Autodesk Fusion 360 part; units mm, degrees
(part 22 of 25)
  line L221 (7.4676, 44.45) -> (8.7884, 44.45)
  arc A279 (8.7884, 33.9598) -> (8.7884, 34.6202) centre (8.7884, 34.29) ccw
  arc A280 (2.3876, 44.7802) -> (2.3876, 44.1198) centre (2.3876, 44.45) ccw
  arc A281 (32.5501, 16.51) -> (33.4899, 16.51) centre (33.02, 16.51) ccw
  arc A282 (8.7884, 44.1198) -> (8.7884, 44.7802) centre (8.7884, 44.45) ccw
  arc A283 (3.7084, 44.1198) -> (3.7084, 44.7802) centre (3.7084, 44.45) ccw
  arc A284 (8.7884, 41.5798) -> (8.7884, 42.2402) centre (8.7884, 41.91) ccw
  arc A285 (3.7084, 41.5798) -> (3.7084, 42.2402) centre (3.7084, 41.91) ccw
  arc A286 (8.7884, 33.9598) -> (8.7884, 34.6202) centre (8.7884, 34.29) ccw
  arc A287 (2.3876, 42.2402) -> (2.3876, 41.5798) centre (2.3876, 41.91) ccw
  line L222 (4.6482, 3.971) -> (4.8936, 4.2164)
  arc A288 (3.7084, 41.5798) -> (3.7084, 42.2402) centre (3.7084, 41.91) ccw
  line L223 (4.6482, 6.511) -> (4.8936, 6.7564)
  line L224 (2.3876, 41.91) -> (3.7084, 41.91)
  line L225 (7.4676, 44.45) -> (8.7884, 44.45)
  arc A289 (7.4676, 42.2402) -> (7.4676, 41.5798) centre (7.4676, 41.91) ccw
  arc A290 (38.5699, 16.51) -> (37.6301, 16.51) centre (38.1, 16.51) ccw
  line L226 (4.8936, 5.9182) -> (4.6482, 6.1636)
  arc A291 (7.4676, 44.7802) -> (7.4676, 44.1198) centre (7.4676, 44.45) ccw
  line L227 (5.4864, 3.6236) -> (5.241, 3.3782)
  arc A292 (8.7884, 44.1198) -> (8.7884, 44.7802) centre (8.7884, 44.45) ccw
  arc A293 (7.4676, 34.6202) -> (7.4676, 33.9598) centre (7.4676, 34.29) ccw
  arc A294 (7.4676, 42.2402) -> (7.4676, 41.5798) centre (7.4676, 41.91) ccw
  arc A295 (8.7884, 41.5798) -> (8.7884, 42.2402) centre (8.7884, 41.91) ccw
  arc A296 (2.3876, 42.2402) -> (2.3876, 41.5798) centre (2.3876, 41.91) ccw
  line L228 (4.6482, 3.6236) -> (4.6482, 3.971)
  line L229 (5.4864, 3.6236) -> (5.241, 3.3782)
  line L230 (5.4864, 3.971) -> (5.4864, 3.6236)
  line L231 (5.241, 5.9182) -> (4.8936, 5.9182)
  line L232 (2.3876, 41.91) -> (3.7084, 41.91)
  line L233 (5.241, 5.9182) -> (4.8936, 5.9182)
  arc A297 (7.4676, 44.7802) -> (7.4676, 44.1198) centre (7.4676, 44.45) ccw
  line L234 (7.4676, 34.29) -> (8.7884, 34.29)
  line L235 (5.241, 6.7564) -> (5.4864, 6.511)
  line L236 (4.8936, 4.2164) -> (5.241, 4.2164)
  line L237 (4.6482, 6.1636) -> (4.6482, 6.511)
  line L238 (4.8936, 5.9182) -> (4.6482, 6.1636)
  arc A298 (41.1099, 16.51) -> (40.1701, 16.51) centre (40.64, 16.51) ccw
  arc A299 (41.1099, 16.51) -> (40.1701, 16.51) centre (40.64, 16.51) ccw
  arc A300 (2.3876, 44.7802) -> (2.3876, 44.1198) centre (2.3876, 44.45) ccw
  arc A301 (2.3876, 34.6202) -> (2.3876, 33.9598) centre (2.3876, 34.29) ccw
  line L239 (7.4676, 34.29) -> (8.7884, 34.29)
  arc A302 (40.1701, 16.51) -> (41.1099, 16.51) centre (40.64, 16.51) ccw
  arc A303 (3.7084, 33.9598) -> (3.7084, 34.6202) centre (3.7084, 34.29) ccw
  line L240 (5.241, 4.2164) -> (5.4864, 3.971)
  line L241 (2.3876, 44.45) -> (3.7084, 44.45)
  arc A304 (36.0299, 16.51) -> (35.0901, 16.51) centre (35.56, 16.51) ccw
  arc A305 (37.6301, 16.51) -> (38.5699, 16.51) centre (38.1, 16.51) ccw
  arc A306 (37.6301, 16.51) -> (38.5699, 16.51) centre (38.1, 16.51) ccw
  arc A307 (38.5699, 16.51) -> (37.6301, 16.51) centre (38.1, 16.51) ccw
  line L242 (2.3876, 34.29) -> (3.7084, 34.29)
  line L243 (2.3876, 34.29) -> (3.7084, 34.29)
  line L244 (4.8936, 6.7564) -> (5.241, 6.7564)
  line L245 (7.4676, 41.91) -> (8.7884, 41.91)
  line L246 (13.5509, 3.9837) -> (13.7963, 4.2291)
  line L247 (4.8936, 3.3782) -> (4.6482, 3.6236)
  line L248 (72.1868, 12.3092) -> (72.1868, 12.5828)
  line L249 (14.1437, 4.2291) -> (14.3891, 3.9837)
  line L250 (72.6538, 12.7762) -> (72.8472, 12.5828)
  line L251 (14.1437, 6.7691) -> (14.3891, 6.5237)
  line L252 (4.8936, 4.2164) -> (5.241, 4.2164)
  line L253 (14.1437, 5.9309) -> (13.7963, 5.9309)
  line L254 (5.4864, 6.1636) -> (5.241, 5.9182)
  line L255 (5.4864, 6.511) -> (5.4864, 6.1636)
  line L256 (13.5509, 6.5237) -> (13.7963, 6.7691)
  line L257 (13.5509, 6.1763) -> (13.5509, 6.5237)
  line L258 (14.3891, 3.6363) -> (14.1437, 3.3909)
  line L259 (72.3802, 12.7762) -> (72.6538, 12.7762)
  line L260 (5.241, 4.2164) -> (5.4864, 3.971)
  line L261 (4.6482, 3.971) -> (4.8936, 4.2164)
  line L262 (4.6482, 6.1636) -> (4.6482, 6.511)
  line L263 (13.7963, 4.2291) -> (14.1437, 4.2291)
  line L264 (14.3891, 6.1763) -> (14.1437, 5.9309)
  line L265 (14.1437, 3.3909) -> (13.7963, 3.3909)
  line L266 (72.6538, 12.7762) -> (72.8472, 12.5828)
  line L267 (5.241, 3.3782) -> (4.8936, 3.3782)
  line L268 (72.8472, 12.5828) -> (72.8472, 12.3092)
  line L269 (13.5509, 3.9837) -> (13.7963, 4.2291)
  line L270 (5.4864, 6.511) -> (5.4864, 6.1636)
  line L271 (4.8936, 3.3782) -> (4.6482, 3.6236)
  line L272 (4.6482, 3.6236) -> (4.6482, 3.971)
  line L273 (4.8936, 4.2164) -> (5.241, 4.2164)
  line L274 (13.7963, 6.7691) -> (14.1437, 6.7691)
  line L275 (14.3891, 6.1763) -> (14.1437, 5.9309)
  line L276 (14.1437, 4.2291) -> (14.3891, 3.9837)
  line L277 (14.1437, 5.9309) -> (13.7963, 5.9309)
  line L278 (72.6538, 12.1158) -> (72.3802, 12.1158)
  line L279 (4.8936, 6.7564) -> (5.241, 6.7564)
  line L280 (13.5509, 3.6363) -> (13.5509, 3.9837)
  line L281 (14.1437, 3.3909) -> (13.7963, 3.3909)
  line L282 (5.4864, 3.971) -> (5.4864, 3.6236)
  line L283 (13.7963, 3.3909) -> (13.5509, 3.6363)
  line L284 (13.5509, 3.6363) -> (13.5509, 3.9837)
  line L285 (4.6482, 6.511) -> (4.8936, 6.7564)
  line L286 (14.3891, 3.9837) -> (14.3891, 3.6363)
  line L287 (14.3891, 3.9837) -> (14.3891, 3.6363)
  line L288 (13.7963, 4.2291) -> (14.1437, 4.2291)
  line L289 (13.5509, 6.1763) -> (13.5509, 6.5237)
  line L290 (72.1868, 12.3092) -> (72.1868, 12.5828)
  line L291 (13.5509, 6.5237) -> (13.7963, 6.7691)
  line L292 (5.4864, 6.1636) -> (5.241, 5.9182)
  line L293 (13.7963, 3.3909) -> (13.5509, 3.6363)
  line L294 (14.3891, 3.6363) -> (14.1437, 3.3909)
  line L295 (14.1437, 6.7691) -> (14.3891, 6.5237)
  line L296 (13.7963, 6.7691) -> (14.1437, 6.7691)
  line L297 (5.241, 3.3782) -> (4.8936, 3.3782)
  line L298 (4.8936, 6.7564) -> (5.241, 6.7564)
  line L299 (13.7963, 5.9309) -> (13.5509, 6.1763)
  line L300 (13.7963, 6.7691) -> (14.1437, 6.7691)
  line L301 (14.3891, 6.5237) -> (14.3891, 6.1763)
  line L302 (13.7963, 4.2291) -> (14.1437, 4.2291)
  line L303 (13.7963, 5.9309) -> (13.5509, 6.1763)
  line L304 (5.241, 6.7564) -> (5.4864, 6.511)
  line L305 (13.7963, 6.7691) -> (14.1437, 6.7691)
  line L306 (4.8936, 4.2164) -> (5.241, 4.2164)
  line L307 (13.7963, 4.2291) -> (14.1437, 4.2291)
  line L308 (14.3891, 6.5237) -> (14.3891, 6.1763)
  line L309 (72.1868, 12.3092) -> (72.1868, 12.5828)
  line L310 (82.5402, 12.7762) -> (82.8138, 12.7762)
  line L311 (4.9686, 11.7475) -> (5.2422, 11.7475)
  line L312 (15.5956, 11.5541) -> (15.5956, 11.2805)
  line L313 (15.5956, 11.5541) -> (15.5956, 11.2805)
  line L314 (72.1868, 12.5828) -> (72.3802, 12.7762)
  line L315 (72.3802, 12.1158) -> (72.1868, 12.3092)
  line L316 (82.5402, 12.7762) -> (82.8138, 12.7762)
  line L317 (15.1286, 11.0871) -> (14.9352, 11.2805)
  line L318 (82.8138, 12.1158) -> (82.5402, 12.1158)
  line L319 (83.0072, 12.5828) -> (83.0072, 12.3092)
  line L320 (15.4022, 11.0871) -> (15.1286, 11.0871)
  line L321 (72.1868, 12.5828) -> (72.3802, 12.7762)
  line L322 (14.9352, 11.5541) -> (15.1286, 11.7475)
  line L323 (4.7752, 11.5541) -> (4.9686, 11.7475)
  line L324 (82.5402, 12.1158) -> (82.3468, 12.3092)
  line L325 (82.3468, 12.5828) -> (82.5402, 12.7762)
  line L326 (83.0072, 12.3092) -> (82.8138, 12.1158)
  line L327 (82.3468, 12.3092) -> (82.3468, 12.5828)
  line L328 (83.0072, 12.5828) -> (83.0072, 12.3092)
  line L329 (82.3468, 12.3092) -> (82.3468, 12.5828)
  line L330 (82.8138, 12.7762) -> (83.0072, 12.5828)
  line L331 (72.1868, 12.3092) -> (72.1868, 12.5828)
  line L332 (15.1286, 11.0871) -> (14.9352, 11.2805)
  line L333 (5.4356, 11.5541) -> (5.4356, 11.2805)
  line L334 (72.6538, 12.1158) -> (72.3802, 12.1158)
  line L335 (4.7752, 11.2805) -> (4.7752, 11.5541)
  line L336 (14.9352, 11.2805) -> (14.9352, 11.5541)
  line L337 (15.5956, 11.2805) -> (15.4022, 11.0871)
  line L338 (4.9686, 11.0871) -> (4.7752, 11.2805)
  line L339 (14.9352, 11.2805) -> (14.9352, 11.5541)
  line L340 (14.9352, 11.5541) -> (15.1286, 11.7475)
  line L341 (15.1286, 11.7475) -> (15.4022, 11.7475)
  line L342 (15.1286, 11.7475) -> (15.4022, 11.7475)
  line L343 (4.7752, 11.2805) -> (4.7752, 11.5541)
  line L344 (83.0072, 12.3092) -> (82.8138, 12.1158)
  line L345 (72.3802, 12.1158) -> (72.1868, 12.3092)
  line L346 (82.3468, 12.3092) -> (82.3468, 12.5828)
  line L347 (82.5402, 12.1158) -> (82.3468, 12.3092)
  line L348 (5.2422, 11.0871) -> (4.9686, 11.0871)
  line L349 (15.5956, 11.5541) -> (15.5956, 11.2805)
  line L350 (4.7752, 11.5541) -> (4.9686, 11.7475)
  line L351 (82.8138, 12.1158) -> (82.5402, 12.1158)
  line L352 (5.4356, 11.5541) -> (5.4356, 11.2805)
  line L353 (72.8472, 12.5828) -> (72.8472, 12.3092)
  line L354 (82.3468, 12.5828) -> (82.5402, 12.7762)
  line L355 (15.5956, 11.2805) -> (15.4022, 11.0871)
  line L356 (5.2422, 11.0871) -> (4.9686, 11.0871)
  line L357 (82.3468, 12.3092) -> (82.3468, 12.5828)
  line L358 (72.8472, 12.3092) -> (72.6538, 12.1158)
  line L359 (72.8472, 12.3092) -> (72.6538, 12.1158)
  line L360 (15.5956, 11.5541) -> (15.5956, 11.2805)
  line L361 (82.8138, 12.7762) -> (83.0072, 12.5828)
  line L362 (15.4022, 11.7475) -> (15.5956, 11.5541)
  line L363 (15.4022, 11.0871) -> (15.1286, 11.0871)
  line L364 (5.4356, 11.2805) -> (5.2422, 11.0871)
  line L365 (72.3802, 12.7762) -> (72.6538, 12.7762)
  line L366 (15.4022, 11.7475) -> (15.5956, 11.5541)
  line L367 (5.4356, 11.5541) -> (5.4356, 11.2805)
  line L368 (72.5268, 25.7302) -> (72.7202, 25.5368)
  line L369 (5.2422, 11.7475) -> (5.4356, 11.5541)
  line L370 (82.8802, 25.5368) -> (82.8802, 25.2632)
  line L371 (72.2532, 25.0698) -> (72.0598, 25.2632)
  line L372 (82.6868, 25.7302) -> (82.8802, 25.5368)
  line L373 (72.7202, 25.5368) -> (72.7202, 25.2632)
  line L374 (82.8802, 25.2632) -> (82.6868, 25.0698)
  line L375 (5.2422, 11.7475) -> (5.4356, 11.5541)
  line L376 (82.4132, 25.0698) -> (82.2198, 25.2632)
  line L377 (72.5268, 25.0698) -> (72.2532, 25.0698)
  line L378 (72.7202, 25.2632) -> (72.5268, 25.0698)
  line L379 (5.4356, 11.2805) -> (5.2422, 11.0871)
  line L380 (82.6868, 25.7302) -> (82.8802, 25.5368)
  line L381 (82.6868, 25.0698) -> (82.4132, 25.0698)
  line L382 (82.2198, 25.5368) -> (82.4132, 25.7302)
  line L383 (82.2198, 25.5368) -> (82.4132, 25.7302)
  line L384 (72.0598, 25.2632) -> (72.0598, 25.5368)
  line L385 (68.2498, 20.1832) -> (68.2498, 20.4568)
  line L386 (58.7502, 20.1832) -> (58.5568, 19.9898)
  line L387 (68.2498, 20.4568) -> (68.4432, 20.6502)
  line L388 (68.4432, 20.6502) -> (68.7168, 20.6502)
  line L389 (72.7202, 25.5368) -> (72.7202, 25.2632)
  line L390 (58.5568, 20.6502) -> (58.7502, 20.4568)
  line L391 (72.0598, 25.2632) -> (72.0598, 25.5368)
  line L392 (72.0598, 25.5368) -> (72.2532, 25.7302)
  line L393 (72.0598, 25.2632) -> (72.0598, 25.5368)
  line L394 (68.9102, 20.1832) -> (68.7168, 19.9898)
  line L395 (58.0898, 20.1832) -> (58.0898, 20.4568)
  line L396 (72.0598, 25.2632) -> (72.0598, 25.5368)
  line L397 (58.2832, 19.9898) -> (58.0898, 20.1832)
  line L398 (72.5268, 25.7302) -> (72.7202, 25.5368)
  line L399 (82.6868, 25.0698) -> (82.4132, 25.0698)
  line L400 (72.2532, 25.7302) -> (72.5268, 25.7302)
  line L401 (72.2532, 25.0698) -> (72.0598, 25.2632)
  line L402 (82.8802, 25.5368) -> (82.8802, 25.2632)
  line L403 (68.2498, 20.4568) -> (68.4432, 20.6502)
  line L404 (68.2498, 20.1832) -> (68.2498, 20.4568)
  line L405 (68.7168, 20.6502) -> (68.9102, 20.4568)
  line L406 (58.5568, 19.9898) -> (58.2832, 19.9898)
  line L407 (58.2832, 20.6502) -> (58.5568, 20.6502)
  line L408 (82.2198, 25.2632) -> (82.2198, 25.5368)
  line L409 (72.7202, 25.2632) -> (72.5268, 25.0698)
  line L410 (82.4132, 25.7302) -> (82.6868, 25.7302)
  line L411 (68.2498, 20.1832) -> (68.2498, 20.4568)
  line L412 (68.4432, 19.9898) -> (68.2498, 20.1832)
  line L413 (58.7502, 20.4568) -> (58.7502, 20.1832)
  line L414 (68.7168, 20.6502) -> (68.9102, 20.4568)
  line L415 (4.9686, 11.0871) -> (4.7752, 11.2805)
  line L416 (5.4356, 11.5541) -> (5.4356, 11.2805)
  line L417 (72.2532, 25.7302) -> (72.5268, 25.7302)
  line L418 (82.2198, 25.2632) -> (82.2198, 25.5368)
  line L419 (82.4132, 25.0698) -> (82.2198, 25.2632)
  line L420 (68.7168, 19.9898) -> (68.4432, 19.9898)
  line L421 (72.5268, 25.0698) -> (72.2532, 25.0698)
  line L422 (58.0898, 20.4568) -> (58.2832, 20.6502)
  line L423 (82.8802, 25.2632) -> (82.6868, 25.0698)
  line L424 (4.9686, 11.7475) -> (5.2422, 11.7475)
  line L425 (68.9102, 20.4568) -> (68.9102, 20.1832)
  line L426 (82.2198, 25.2632) -> (82.2198, 25.5368)
  line L427 (82.4132, 25.7302) -> (82.6868, 25.7302)
  line L428 (72.0598, 25.5368) -> (72.2532, 25.7302)
  line L429 (58.2832, 19.9898) -> (58.0898, 20.1832)
  line L430 (58.0898, 20.1832) -> (58.0898, 20.4568)
  line L431 (82.2198, 25.2632) -> (82.2198, 25.5368)
  line L432 (58.2832, 25.7302) -> (58.5568, 25.7302)
  line L433 (68.9102, 25.2632) -> (68.7168, 25.0698)
  line L434 (68.2498, 25.5368) -> (68.4432, 25.7302)
  line L435 (58.0898, 25.5368) -> (58.2832, 25.7302)
  line L436 (58.0898, 20.1832) -> (58.0898, 20.4568)
  line L437 (58.7502, 25.5368) -> (58.7502, 25.2632)
  line L438 (58.7502, 20.4568) -> (58.7502, 20.1832)
  line L439 (58.0898, 25.2632) -> (58.0898, 25.5368)
  line L440 (68.9102, 20.1832) -> (68.7168, 19.9898)
  line L441 (58.7502, 25.5368) -> (58.7502, 25.2632)
  line L442 (58.7502, 25.5368) -> (58.7502, 25.2632)
  line L443 (40.9702, 37.9632) -> (40.7768, 37.7698)
  line L444 (58.2832, 25.7302) -> (58.5568, 25.7302)
  line L445 (50.6632, 38.4302) -> (50.9368, 38.4302)
  line L446 (68.9102, 25.5368) -> (68.9102, 25.2632)
  line L447 (68.9102, 25.2632) -> (68.7168, 25.0698)
  line L448 (50.9368, 37.7698) -> (50.6632, 37.7698)
  line L449 (40.7768, 38.4302) -> (40.9702, 38.2368)
  line L450 (51.1302, 38.2368) -> (51.1302, 37.9632)
  line L451 (50.4698, 37.9632) -> (50.4698, 38.2368)
  line L452 (40.9702, 38.2368) -> (40.9702, 37.9632)
  line L453 (40.7768, 37.7698) -> (40.5032, 37.7698)
  line L454 (68.9102, 25.5368) -> (68.9102, 25.2632)
  line L455 (68.2498, 25.5368) -> (68.4432, 25.7302)
  line L456 (58.5568, 25.7302) -> (58.7502, 25.5368)
  line L457 (58.0898, 20.4568) -> (58.2832, 20.6502)
  line L458 (50.9368, 38.4302) -> (51.1302, 38.2368)
  line L459 (58.5568, 19.9898) -> (58.2832, 19.9898)
  line L460 (40.7768, 37.7698) -> (40.5032, 37.7698)
  line L461 (58.5568, 25.0698) -> (58.2832, 25.0698)
  line L462 (68.7168, 19.9898) -> (68.4432, 19.9898)
  line L463 (40.5032, 37.7698) -> (40.3098, 37.9632)
  line L464 (40.5032, 38.4302) -> (40.7768, 38.4302)
  line L465 (40.3098, 37.9632) -> (40.3098, 38.2368)
  line L466 (58.2832, 25.0698) -> (58.0898, 25.2632)
  line L467 (68.2498, 25.2632) -> (68.2498, 25.5368)
  line L468 (50.6632, 38.4302) -> (50.9368, 38.4302)
  line L469 (68.9102, 25.5368) -> (68.9102, 25.2632)
  line L470 (68.7168, 25.0698) -> (68.4432, 25.0698)
  line L471 (68.7168, 25.0698) -> (68.4432, 25.0698)
  line L472 (68.7168, 25.7302) -> (68.9102, 25.5368)
  line L473 (58.7502, 20.1832) -> (58.5568, 19.9898)
  line L474 (58.2832, 20.6502) -> (58.5568, 20.6502)
  line L475 (58.0898, 25.5368) -> (58.2832, 25.7302)
  line L476 (68.4432, 25.7302) -> (68.7168, 25.7302)
  line L477 (58.7502, 25.5368) -> (58.7502, 25.2632)
  line L478 (68.9102, 20.4568) -> (68.9102, 20.1832)
  line L479 (68.4432, 20.6502) -> (68.7168, 20.6502)
  line L480 (58.0898, 25.2632) -> (58.0898, 25.5368)
  line L481 (68.2498, 25.2632) -> (68.2498, 25.5368)
  line L482 (68.4432, 25.7302) -> (68.7168, 25.7302)
  line L483 (58.5568, 25.7302) -> (58.7502, 25.5368)
  line L484 (68.4432, 25.0698) -> (68.2498, 25.2632)
  line L485 (58.2832, 25.0698) -> (58.0898, 25.2632)
  line L486 (58.7502, 25.2632) -> (58.5568, 25.0698)
  line L487 (58.5568, 25.0698) -> (58.2832, 25.0698)
  line L488 (68.9102, 25.5368) -> (68.9102, 25.2632)
  line L489 (58.7502, 25.2632) -> (58.5568, 25.0698)
  line L490 (68.4432, 19.9898) -> (68.2498, 20.1832)
  line L491 (68.2498, 20.1832) -> (68.2498, 20.4568)
  line L492 (58.0898, 20.1832) -> (58.0898, 20.4568)
  line L493 (58.5568, 20.6502) -> (58.7502, 20.4568)
  line L494 (68.4432, 25.0698) -> (68.2498, 25.2632)
  line L495 (68.7168, 25.7302) -> (68.9102, 25.5368)
  line L496 (51.1302, 42.0468) -> (51.1302, 41.7732)
  line L497 (50.9368, 42.2402) -> (51.1302, 42.0468)
  line L498 (40.7768, 42.2402) -> (40.9702, 42.0468)
  line L499 (50.6632, 37.7698) -> (50.4698, 37.9632)
  line L500 (40.3098, 41.7732) -> (40.3098, 42.0468)
  line L501 (51.1302, 41.7732) -> (50.9368, 41.5798)
  line L502 (51.1302, 41.7732) -> (50.9368, 41.5798)
  line L503 (40.9702, 37.9632) -> (40.7768, 37.7698)
  line L504 (40.9702, 38.2368) -> (40.9702, 37.9632)
  line L505 (50.9368, 38.4302) -> (51.1302, 38.2368)
  line L506 (50.9368, 42.2402) -> (51.1302, 42.0468)
  line L507 (40.7768, 41.5798) -> (40.5032, 41.5798)
  line L508 (50.9368, 41.5798) -> (50.6632, 41.5798)
  line L509 (40.9702, 41.7732) -> (40.7768, 41.5798)
  line L510 (50.6632, 37.7698) -> (50.4698, 37.9632)
  line L511 (50.4698, 38.2368) -> (50.6632, 38.4302)
  line L512 (40.3098, 38.2368) -> (40.5032, 38.4302)
  line L513 (51.1302, 37.9632) -> (50.9368, 37.7698)
  line L514 (40.5032, 42.2402) -> (40.7768, 42.2402)
  line L515 (40.9702, 42.0468) -> (40.9702, 41.7732)
  line L516 (36.4998, 41.7732) -> (36.4998, 42.0468)
  line L517 (50.4698, 37.9632) -> (50.4698, 38.2368)
  line L518 (36.4998, 41.7732) -> (36.4998, 42.0468)
  line L519 (40.9702, 42.0468) -> (40.9702, 41.7732)
  line L520 (40.9702, 38.2368) -> (40.9702, 37.9632)
  line L521 (40.5032, 38.4302) -> (40.7768, 38.4302)
  line L522 (51.1302, 38.2368) -> (51.1302, 37.9632)
  line L523 (50.9368, 37.7698) -> (50.6632, 37.7698)
  line L524 (40.5032, 42.2402) -> (40.7768, 42.2402)
  line L525 (40.7768, 42.2402) -> (40.9702, 42.0468)
  line L526 (50.6632, 42.2402) -> (50.9368, 42.2402)
  line L527 (26.3398, 42.0468) -> (26.5332, 42.2402)
  line L528 (37.1602, 41.7732) -> (36.9668, 41.5798)
  line L529 (50.4698, 38.2368) -> (50.6632, 38.4302)
  line L530 (40.3098, 42.0468) -> (40.5032, 42.2402)
  line L531 (40.9702, 41.7732) -> (40.7768, 41.5798)
  line L532 (51.1302, 42.0468) -> (51.1302, 41.7732)
  line L533 (51.1302, 38.2368) -> (51.1302, 37.9632)
  line L534 (40.5032, 41.5798) -> (40.3098, 41.7732)
  line L535 (50.4698, 41.7732) -> (50.4698, 42.0468)
  line L536 (50.6632, 41.5798) -> (50.4698, 41.7732)
  line L537 (40.7768, 41.5798) -> (40.5032, 41.5798)
  line L538 (50.4698, 41.7732) -> (50.4698, 42.0468)
  line L539 (36.9668, 41.5798) -> (36.6932, 41.5798)
  line L540 (40.3098, 41.7732) -> (40.3098, 42.0468)
  line L541 (26.5332, 41.5798) -> (26.3398, 41.7732)
  line L542 (50.4698, 42.0468) -> (50.6632, 42.2402)
  line L543 (51.1302, 37.9632) -> (50.9368, 37.7698)
  line L544 (50.4698, 41.7732) -> (50.4698, 42.0468)
  line L545 (40.7768, 38.4302) -> (40.9702, 38.2368)
  line L546 (50.4698, 42.0468) -> (50.6632, 42.2402)
  line L547 (50.4698, 41.7732) -> (50.4698, 42.0468)
  line L548 (51.1302, 38.2368) -> (51.1302, 37.9632)
  line L549 (40.9702, 38.2368) -> (40.9702, 37.9632)
  line L550 (40.3098, 41.7732) -> (40.3098, 42.0468)
  line L551 (40.3098, 41.7732) -> (40.3098, 42.0468)
  line L552 (40.5032, 41.5798) -> (40.3098, 41.7732)
  line L553 (50.6632, 41.5798) -> (50.4698, 41.7732)
  line L554 (40.3098, 42.0468) -> (40.5032, 42.2402)
  line L555 (40.3098, 37.9632) -> (40.3098, 38.2368)
  line L556 (50.6632, 42.2402) -> (50.9368, 42.2402)
  line L557 (40.5032, 37.7698) -> (40.3098, 37.9632)
  line L558 (50.9368, 41.5798) -> (50.6632, 41.5798)
  line L559 (40.3098, 38.2368) -> (40.5032, 38.4302)
  line L560 (36.9668, 41.5798) -> (36.6932, 41.5798)
  line L561 (36.4998, 42.0468) -> (36.6932, 42.2402)
  line L562 (4.7498, 15.1032) -> (4.7498, 15.3768)
  line L563 (15.5702, 15.3768) -> (15.5702, 15.1032)
  line L564 (26.8068, 42.2402) -> (27.0002, 42.0468)
  line L565 (5.4102, 15.1032) -> (5.2168, 14.9098)
  line L566 (26.5332, 42.2402) -> (26.8068, 42.2402)
  line L567 (5.2168, 14.9098) -> (4.9432, 14.9098)
  line L568 (26.8068, 42.2402) -> (27.0002, 42.0468)
  line L569 (26.3398, 41.7732) -> (26.3398, 42.0468)
  line L570 (15.3768, 14.9098) -> (15.1032, 14.9098)
  line L571 (15.5702, 15.3768) -> (15.5702, 15.1032)
  line L572 (15.1032, 15.5702) -> (15.3768, 15.5702)
  line L573 (15.3768, 15.5702) -> (15.5702, 15.3768)
  line L574 (26.5332, 42.2402) -> (26.8068, 42.2402)
  line L575 (15.1032, 14.9098) -> (14.9098, 15.1032)
  line L576 (15.3768, 14.9098) -> (15.1032, 14.9098)
  line L577 (4.9432, 15.5702) -> (5.2168, 15.5702)
  line L578 (14.9098, 15.3768) -> (15.1032, 15.5702)
  line L579 (14.9098, 15.3768) -> (15.1032, 15.5702)
  line L580 (15.3768, 15.5702) -> (15.5702, 15.3768)
  line L581 (15.5702, 15.3768) -> (15.5702, 15.1032)
  line L582 (5.4102, 15.3768) -> (5.4102, 15.1032)
  line L583 (5.2168, 14.9098) -> (4.9432, 14.9098)
  line L584 (4.9432, 14.9098) -> (4.7498, 15.1032)
  line L585 (5.2168, 15.5702) -> (5.4102, 15.3768)
  line L586 (5.4102, 15.3768) -> (5.4102, 15.1032)
  line L587 (36.6932, 42.2402) -> (36.9668, 42.2402)
  line L588 (4.7498, 15.3768) -> (4.9432, 15.5702)
  line L589 (27.0002, 41.7732) -> (26.8068, 41.5798)
  line L590 (26.3398, 41.7732) -> (26.3398, 42.0468)
  line L591 (5.4102, 15.3768) -> (5.4102, 15.1032)
  line L592 (4.7498, 15.1032) -> (4.7498, 15.3768)
  line L593 (15.5702, 15.1032) -> (15.3768, 14.9098)
  line L594 (27.0002, 42.0468) -> (27.0002, 41.7732)
  line L595 (36.4998, 42.0468) -> (36.6932, 42.2402)
  line L596 (15.1032, 15.5702) -> (15.3768, 15.5702)
  line L597 (14.9098, 15.1032) -> (14.9098, 15.3768)
  line L598 (37.1602, 42.0468) -> (37.1602, 41.7732)
  line L599 (15.5702, 15.1032) -> (15.3768, 14.9098)
  line L600 (26.3398, 41.7732) -> (26.3398, 42.0468)
  line L601 (26.8068, 41.5798) -> (26.5332, 41.5798)
  line L602 (36.4998, 41.7732) -> (36.4998, 42.0468)
  line L603 (4.7498, 15.3768) -> (4.9432, 15.5702)
  line L604 (5.4102, 15.1032) -> (5.2168, 14.9098)
  line L605 (26.8068, 41.5798) -> (26.5332, 41.5798)
  line L606 (36.4998, 41.7732) -> (36.4998, 42.0468)
  line L607 (27.0002, 41.7732) -> (26.8068, 41.5798)
  line L608 (26.3398, 41.7732) -> (26.3398, 42.0468)
  line L609 (36.6932, 41.5798) -> (36.4998, 41.7732)
  line L610 (36.6932, 42.2402) -> (36.9668, 42.2402)
  line L611 (36.9668, 42.2402) -> (37.1602, 42.0468)
  line L612 (36.6932, 41.5798) -> (36.4998, 41.7732)
  line L613 (27.0002, 42.0468) -> (27.0002, 41.7732)
  line L614 (37.1602, 42.0468) -> (37.1602, 41.7732)
  line L615 (15.5702, 15.3768) -> (15.5702, 15.1032)
  line L616 (14.9098, 15.1032) -> (14.9098, 15.3768)
  line L617 (5.2168, 15.5702) -> (5.4102, 15.3768)
  line L618 (36.9668, 42.2402) -> (37.1602, 42.0468)
  line L619 (37.1602, 41.7732) -> (36.9668, 41.5798)
  line L620 (26.3398, 42.0468) -> (26.5332, 42.2402)
  line L621 (26.5332, 41.5798) -> (26.3398, 41.7732)
  line L622 (15.1032, 14.9098) -> (14.9098, 15.1032)
  line L623 (4.9432, 14.9098) -> (4.7498, 15.1032)
  arc A308 (74.2188, 21.7805) -> (74.2188, 20.8407) centre (74.2188, 21.3106) ccw
  arc A309 (80.7491, 6.9342) -> (80.7491, 7.874) centre (80.7491, 7.4041) ccw
  arc A310 (74.2188, 16.3195) -> (74.2188, 17.2593) centre (74.2188, 16.7894) ccw
  arc A311 (80.7491, 7.874) -> (80.7491, 6.9342) centre (80.7491, 7.4041) ccw
  line L624 (7.8831, 28.575) -> (7.3569, 28.575)
  line L625 (7.8831, 29.845) -> (8.255, 29.4731)
  line L626 (8.255, 29.4731) -> (8.255, 28.9469)
  arc A312 (80.7491, 7.874) -> (80.7491, 6.9342) centre (80.7491, 7.4041) ccw
  arc A313 (80.7212, 17.2593) -> (80.7212, 16.3195) centre (80.7212, 16.7894) ccw
  line L627 (6.985, 28.9469) -> (6.985, 29.4731)
  line L628 (7.3569, 29.845) -> (7.8831, 29.845)
  line L629 (6.985, 21.3269) -> (6.985, 21.8531)
  arc A314 (80.7491, 2.413) -> (80.7491, 3.3528) centre (80.7491, 2.8829) ccw
  line L630 (7.3569, 28.575) -> (6.985, 28.9469)
  arc A315 (80.7212, 16.3195) -> (80.7212, 17.2593) centre (80.7212, 16.7894) ccw
  line L631 (6.985, 28.9469) -> (6.985, 29.4731)
  line L632 (8.255, 21.8531) -> (8.255, 21.3269)
  arc A316 (74.2467, 6.9342) -> (74.2467, 7.874) centre (74.2467, 7.4041) ccw
  arc A317 (80.7212, 20.8407) -> (80.7212, 21.7805) centre (80.7212, 21.3106) ccw
  arc A318 (74.2467, 2.413) -> (74.2467, 3.3528) centre (74.2467, 2.8829) ccw
  arc A319 (74.2188, 20.8407) -> (74.2188, 21.7805) centre (74.2188, 21.3106) ccw
  arc A320 (80.7491, 3.3528) -> (80.7491, 2.413) centre (80.7491, 2.8829) ccw
  arc A321 (80.7212, 20.8407) -> (80.7212, 21.7805) centre (80.7212, 21.3106) ccw
  arc A322 (74.2188, 20.8407) -> (74.2188, 21.7805) centre (74.2188, 21.3106) ccw
  arc A323 (74.2188, 17.2593) -> (74.2188, 16.3195) centre (74.2188, 16.7894) ccw
  arc A324 (74.2188, 17.2593) -> (74.2188, 16.3195) centre (74.2188, 16.7894) ccw
  arc A325 (80.7212, 17.2593) -> (80.7212, 16.3195) centre (80.7212, 16.7894) ccw
  line L633 (4.9432, 15.5702) -> (5.2168, 15.5702)
  arc A326 (74.2467, 7.874) -> (74.2467, 6.9342) centre (74.2467, 7.4041) ccw
  arc A327 (74.2467, 6.9342) -> (74.2467, 7.874) centre (74.2467, 7.4041) ccw
  arc A328 (80.7491, 6.9342) -> (80.7491, 7.874) centre (80.7491, 7.4041) ccw
  arc A329 (80.7212, 21.7805) -> (80.7212, 20.8407) centre (80.7212, 21.3106) ccw
  line L634 (7.8831, 29.845) -> (8.255, 29.4731)
  arc A330 (80.7491, 3.3528) -> (80.7491, 2.413) centre (80.7491, 2.8829) ccw
  arc A331 (80.7212, 21.7805) -> (80.7212, 20.8407) centre (80.7212, 21.3106) ccw
  line L635 (8.255, 29.4731) -> (8.255, 28.9469)
  line L636 (8.255, 28.9469) -> (7.8831, 28.575)
  line L637 (7.8831, 28.575) -> (7.3569, 28.575)
  line L638 (8.255, 28.9469) -> (7.8831, 28.575)
  line L639 (7.3569, 29.845) -> (7.8831, 29.845)
  line L640 (8.255, 21.3269) -> (7.8831, 20.955)
  line L641 (5.4102, 15.3768) -> (5.4102, 15.1032)
  arc A332 (74.2188, 16.3195) -> (74.2188, 17.2593) centre (74.2188, 16.7894) ccw
  line L642 (7.8831, 28.575) -> (7.3569, 28.575)
  line L643 (6.985, 21.8531) -> (7.3569, 22.225)
  arc A333 (80.7491, 2.413) -> (80.7491, 3.3528) centre (80.7491, 2.8829) ccw
  arc A334 (74.2467, 2.413) -> (74.2467, 3.3528) centre (74.2467, 2.8829) ccw
  line L644 (7.8831, 20.955) -> (7.3569, 20.955)
  line L645 (7.8831, 22.225) -> (8.255, 21.8531)
  line L646 (7.8831, 28.575) -> (7.3569, 28.575)
  line L647 (8.255, 21.8531) -> (8.255, 21.3269)
  arc A335 (74.2467, 7.874) -> (74.2467, 6.9342) centre (74.2467, 7.4041) ccw
  line L648 (6.985, 29.4731) -> (7.3569, 29.845)
  line L649 (8.255, 21.3269) -> (7.8831, 20.955)
  line L650 (7.3569, 20.955) -> (6.985, 21.3269)
  line L651 (7.3569, 28.575) -> (6.985, 28.9469)
  arc A336 (74.2467, 3.3528) -> (74.2467, 2.413) centre (74.2467, 2.8829) ccw
  arc A337 (80.7212, 16.3195) -> (80.7212, 17.2593) centre (80.7212, 16.7894) ccw
  arc A338 (74.2188, 21.7805) -> (74.2188, 20.8407) centre (74.2188, 21.3106) ccw
  line L652 (6.985, 29.4731) -> (7.3569, 29.845)
  arc A339 (74.2467, 3.3528) -> (74.2467, 2.413) centre (74.2467, 2.8829) ccw
  line L653 (7.8831, 20.955) -> (7.3569, 20.955)
  line L654 (6.985, 21.3269) -> (6.985, 21.8531)
  line L655 (7.3569, 22.225) -> (7.8831, 22.225)
  arc A340 (20.9804, 37.7698) -> (20.9804, 38.4302) centre (20.9804, 38.1) ccw
  line L656 (7.8831, 20.955) -> (7.3569, 20.955)
  arc A341 (20.9804, 37.7698) -> (20.9804, 38.4302) centre (20.9804, 38.1) ccw
  line L657 (20.9804, 38.1) -> (19.6596, 38.1)
  line L658 (20.9804, 40.64) -> (19.6596, 40.64)
  arc A342 (19.6596, 43.5102) -> (19.6596, 42.8498) centre (19.6596, 43.18) ccw
  line L659 (7.3569, 20.955) -> (6.985, 21.3269)
  arc A343 (20.9804, 40.3098) -> (20.9804, 40.9702) centre (20.9804, 40.64) ccw
  line L660 (20.9804, 43.18) -> (19.6596, 43.18)
  arc A344 (20.9804, 42.8498) -> (20.9804, 43.5102) centre (20.9804, 43.18) ccw
  arc A345 (20.9804, 40.3098) -> (20.9804, 40.9702) centre (20.9804, 40.64) ccw
  line L661 (7.8831, 20.955) -> (7.3569, 20.955)
  arc A346 (19.6596, 43.5102) -> (19.6596, 42.8498) centre (19.6596, 43.18) ccw
  line L662 (20.9804, 38.1) -> (19.6596, 38.1)
  arc A347 (19.6596, 38.4302) -> (19.6596, 37.7698) centre (19.6596, 38.1) ccw
  arc A348 (19.6596, 38.4302) -> (19.6596, 37.7698) centre (19.6596, 38.1) ccw
  line L663 (7.8831, 22.225) -> (8.255, 21.8531)
  arc A349 (19.6596, 40.9702) -> (19.6596, 40.3098) centre (19.6596, 40.64) ccw
  arc A350 (19.6596, 40.9702) -> (19.6596, 40.3098) centre (19.6596, 40.64) ccw
  line L664 (7.3569, 22.225) -> (7.8831, 22.225)
  line L665 (6.985, 21.8531) -> (7.3569, 22.225)
  line L666 (20.9804, 40.64) -> (19.6596, 40.64)
  arc A351 (20.9804, 42.8498) -> (20.9804, 43.5102) centre (20.9804, 43.18) ccw
  line L667 (20.9804, 43.18) -> (19.6596, 43.18)
  line L668 (10.9601, 50.4698) -> (10.9601, 48.5902)
  line L669 (11.8999, 48.5902) -> (11.8999, 50.4698)
  line L670 (13.5001, 50.4698) -> (13.5001, 48.5902)
  line L671 (14.4399, 48.5902) -> (14.4399, 50.4698)
  line L672 (16.0401, 50.4698) -> (16.0401, 48.5902)
  line L673 (16.9799, 50.4698) -> (16.9799, 48.5902)
  line L674 (18.5801, 48.5902) -> (18.5801, 50.4698)
  line L675 (19.5199, 50.4698) -> (19.5199, 48.5902)
  line L676 (21.1201, 48.5902) -> (21.1201, 50.4698)
  line L677 (22.0599, 50.4698) -> (22.0599, 48.5902)
  line L678 (20.9804, 43.5102) -> (19.6596, 43.5102)
  line L679 (19.6596, 42.8498) -> (20.9804, 42.8498)
  line L680 (20.9804, 40.9702) -> (19.6596, 40.9702)
  line L681 (19.6596, 40.3098) -> (20.9804, 40.3098)
  line L682 (20.9804, 38.4302) -> (19.6596, 38.4302)
  line L683 (19.6596, 37.7698) -> (20.9804, 37.7698)
  line L684 (3.7084, 44.7802) -> (2.3876, 44.7802)
  line L685 (2.3876, 44.1198) -> (3.7084, 44.1198)
  line L686 (7.4676, 44.7802) -> (8.7884, 44.7802)
  line L687 (8.7884, 44.1198) -> (7.4676, 44.1198)
  line L688 (7.4676, 42.2402) -> (8.7884, 42.2402)
  line L689 (8.7884, 41.5798) -> (7.4676, 41.5798)
  line L690 (3.7084, 42.2402) -> (2.3876, 42.2402)
  line L691 (2.3876, 41.5798) -> (3.7084, 41.5798)
  line L692 (2.3876, 34.6202) -> (3.7084, 34.6202)
  line L693 (3.7084, 33.9598) -> (2.3876, 33.9598)
  line L694 (8.7884, 34.6202) -> (7.4676, 34.6202)
  line L695 (7.4676, 33.9598) -> (8.7884, 33.9598)
  line L696 (26.2001, 26.3398) -> (26.2001, 24.4602)
  line L697 (27.1399, 26.3398) -> (27.1399, 24.4602)
  line L698 (28.7401, 26.3398) -> (28.7401, 24.4602)
  line L699 (29.6799, 26.3398) -> (29.6799, 24.4602)
  line L700 (31.2801, 24.4602) -> (31.2801, 26.3398)
  line L701 (32.2199, 26.3398) -> (32.2199, 24.4602)
  line L702 (33.8201, 24.4602) -> (33.8201, 26.3398)
  line L703 (34.7599, 26.3398) -> (34.7599, 24.4602)
  line L704 (36.3601, 24.4602) -> (36.3601, 26.3398)
  line L705 (37.2999, 26.3398) -> (37.2999, 24.4602)
  line L706 (47.7901, 26.3398) -> (47.7901, 24.4602)
  line L707 (48.7299, 24.4602) -> (48.7299, 26.3398)
  line L708 (50.3301, 26.3398) -> (50.3301, 24.4602)
  line L709 (51.2699, 24.4602) -> (51.2699, 26.3398)
  line L710 (52.8701, 26.3398) -> (52.8701, 24.4602)
  line L711 (53.8099, 24.4602) -> (53.8099, 26.3398)
  line L712 (60.4901, 30.8102) -> (60.4901, 32.6898)
  line L713 (61.4299, 30.8102) -> (61.4299, 32.6898)
  line L714 (63.0301, 32.6898) -> (63.0301, 30.8102)
  line L715 (63.9699, 30.8102) -> (63.9699, 32.6898)
  line L716 (65.5701, 32.6898) -> (65.5701, 30.8102)
  line L717 (66.5099, 30.8102) -> (66.5099, 32.6898)
  line L718 (73.1901, 32.6898) -> (73.1901, 30.8102)
  line L719 (74.1299, 30.8102) -> (74.1299, 32.6898)
  line L720 (75.7301, 32.6898) -> (75.7301, 30.8102)
  line L721 (76.6699, 30.8102) -> (76.6699, 32.6898)
  line L722 (78.2701, 32.6898) -> (78.2701, 30.8102)
  line L723 (79.2099, 30.8102) -> (79.2099, 32.6898)
  line L724 (80.8101, 32.6898) -> (80.8101, 30.8102)
  line L725 (81.7499, 30.8102) -> (81.7499, 32.6898)
  line L726 (57.9501, 44.1198) -> (57.9501, 42.2402)
  line L727 (58.8899, 42.2402) -> (58.8899, 44.1198)
  line L728 (60.4901, 44.1198) -> (60.4901, 42.2402)
  line L729 (61.4299, 42.2402) -> (61.4299, 44.1198)
  line L730 (63.0301, 44.1198) -> (63.0301, 42.2402)
  line L731 (63.9699, 42.2402) -> (63.9699, 44.1198)
  line L732 (65.5701, 44.1198) -> (65.5701, 42.2402)
  line L733 (66.5099, 42.2402) -> (66.5099, 44.1198)
  line L734 (73.1901, 45.3898) -> (73.1901, 43.5102)
  line L735 (74.1299, 43.5102) -> (74.1299, 45.3898)
  line L736 (75.7301, 45.3898) -> (75.7301, 43.5102)
  line L737 (76.6699, 43.5102) -> (76.6699, 45.3898)
  line L738 (79.2099, 45.3898) -> (79.2099, 43.5102)
  line L739 (78.2701, 43.5102) -> (78.2701, 45.3898)
  line L740 (80.8101, 45.3898) -> (80.8101, 43.5102)
  line L741 (81.7499, 43.5102) -> (81.7499, 45.3898)
  constraint tangent A238 L668
  constraint tangent A222 L669
  constraint tangent A226 L670
  constraint tangent A221 L671
  constraint tangent A236 L672
  constraint tangent A231 L673
  constraint tangent A217 L674
  constraint tangent A225 L675
  constraint tangent A224 L676
  constraint tangent A237 L677
  constraint tangent A346 L678
  constraint tangent A344 L679
  constraint tangent A349 L680
  constraint tangent A350 L681
  constraint parallel L680 L681
  constraint tangent A347 L682
  constraint tangent A341 L683
  constraint tangent A280 L684
  constraint tangent A283 L685
  constraint tangent A292 L686
  constraint tangent A297 L687
  constraint tangent A295 L688
  constraint tangent A289 L689
  constraint tangent A296 L690
  constraint tangent A288 L691
  constraint tangent A303 L692
  constraint tangent A301 L693
  constraint tangent A293 L694
  constraint tangent A286 L695
  constraint tangent A153 L696
  constraint tangent A100 L697
  constraint tangent A136 L698
  constraint tangent A136 L699
  constraint tangent A151 L700
  constraint tangent A154 L701
  constraint tangent A152 L702
  constraint tangent A152 L703
  constraint tangent A149 L704
  constraint tangent A147 L705
  constraint tangent A252 L706
  constraint tangent A264 L707
  constraint tangent A257 L708
  constraint tangent A249 L709
  constraint tangent A268 L710
  constraint tangent A266 L711
  constraint tangent A213 L712
  constraint tangent A213 L713
  constraint tangent A198 L714
  constraint tangent A229 L715
  constraint tangent A218 L716
  constraint tangent A218 L717
  constraint tangent A163 L718
  constraint tangent A180 L719
  constraint tangent A168 L720
  constraint tangent A170 L721
  constraint tangent A208 L722
  constraint tangent A208 L723
  constraint tangent A206 L724
  constraint tangent A186 L725
  constraint tangent A209 L726
  constraint tangent A209 L727
  constraint tangent A187 L728
  constraint tangent A204 L729
  constraint tangent A195 L730
  constraint tangent A194 L731
  constraint tangent A185 L732
  constraint tangent A191 L733
  constraint tangent A160 L734
  constraint tangent A169 L735
  constraint tangent A176 L736
  constraint tangent A166 L737
  constraint tangent A181 L738
  constraint tangent A159 L739
  constraint tangent A162 L740
  constraint tangent A158 L741